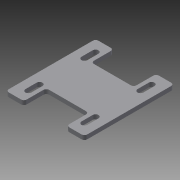
# Autodesk Inventor part: torchMount_back
Saved by Autodesk Inventor 2013 (Build 170138000, 138)
## iProperties
Created: 2012-12-09
Part Number: torchMount_back
Material: Generic
Document SubType Name: Modeling
Designer: Istvan
Density: 1 g/cm^3
Mass: 23.2109 g
Surface Area: 130.889 cm^2
Volume: 23.2109 cm^3
Author: Istvan
Autodesk Inventor part; units mm, degrees
ref_plane "YZ Plane" through (0, 0, 0) normal (1, 0, 0) x (0, 1, 0)
ref_plane "XZ Plane" through (0, 0, 0) normal (0, 1, 0) x (-1, 0, 0)
ref_plane "XY Plane" through (0, 0, 0) normal (0, 0, 1) x (1, 0, 0)
sketch "Sketch1" plane through (0, 0, 0) normal (0, 1, 0) x (-1, 0, 0)
  line L0 (0, 0) -> (20.32, 0)
  line L1 (0, 101.6) -> (0, 0)
  line L2 (44.45, 76.2) -> (20.32, 76.2)
  line L3 (20.32, 76.2) -> (20.32, 101.6)
  line L4 (44.45, 76.2) -> (44.45, 25.4)
  line L5 (20.32, 101.6) -> (0, 101.6)
  line L6 (16.002, 88.9) -> (16.002, 76.2)
  line L7 (9.398, 76.2) -> (9.398, 88.9)
  arc A0 (16.002, 88.9) -> (9.398, 88.9) centre (12.7, 88.9) ccw
  arc A1 (9.398, 76.2) -> (16.002, 76.2) centre (12.7, 76.2) ccw
  line L8 (16.002, 25.4) -> (16.002, 12.7)
  line L9 (9.398, 12.7) -> (9.398, 25.4)
  arc A2 (16.002, 25.4) -> (9.398, 25.4) centre (12.7, 25.4) ccw
  arc A3 (9.398, 12.7) -> (16.002, 12.7) centre (12.7, 12.7) ccw
  line L10 (44.45, 25.4) -> (20.32, 25.4)
  line L11 (20.32, 25.4) -> (20.32, 0)
  dimension "d1" = 101.6
  dimension "d8" = 44.45
  dimension "d11" = 6.604
  dimension "d14" = 12.7
  dimension "d15" = 12.7
  dimension "d18" = 12.7
  dimension "d19" = 20.32
  dimension "d21" = 31.75
  dimension "d23" = 50.8
  dimension "d24" = 25.4
  dimension "d25" = 63.5
  dimension "d26" = 6.604
  constraints: 24 end point, 8 point on circle, 8 tangent, 4 centre point, 4 parallel, 2 vertical, 2 vertical alignment, 1 collinear, 1 horizontal, 1 perpendicular
  measures "d1" distance of L1.start L0.start
  measures "d8" distance between parallel lines of L4 L1
  measures "d11" distance between parallel lines of L6 L7
  measures "d14" distance of A1.centre A0.centre
  measures "d15" distance from line of L5 A0.centre
  measures "d18" distance from line of L0 A3.centre
  measures "d19" distance between parallel lines of L3 L1
  measures "d21" distance from line of L4 A0.centre
  measures "d23" distance between parallel lines of L10 L2
  measures "d24" distance between parallel lines of L10 L0
  measures "d25" distance of A2.centre A0.centre
  measures "d26" distance between parallel lines of L8 L9
extrude "Extrusion1" add sketch "Sketch1" against normal blind 4.7625
fillet "Fillet1" radius 3.175 6 edges at (-20.32, -2.3813, 76.2) (-20.32, -2.3813, 101.6) (0, -2.3813, 101.6) (0, -2.3813, 0) (-20.32, -2.3813, 0) (-20.32, -2.3813, 25.4)
mirror "Mirror2" about plane through (-44.45, 0, 76.2) normal (-1, 0, 0)
equation "\"d26\" = d11"
body "Solid1"
